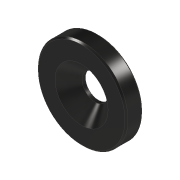
# Autodesk Inventor part: ring wiel
Saved by Autodesk Inventor 2020.3 (Build 243373000, 373)
## iProperties
Created: 2020-09-10
Part Number: ring wiel
Material: Stainless Steel
Document SubType Name: Modeling
Designer: Svend
Density: 8 g/cm^3
Appearance: Semi-Polished
Author: Svend
Autodesk Inventor part; units mm, degrees
ref_plane "YZ Plane" through (0, 0, 0) normal (1, 0, 0) x (0, 1, 0)
ref_plane "XZ Plane" through (0, 0, 0) normal (0, 1, 0) x (-1, 0, 0)
ref_plane "XY Plane" through (0, 0, 0) normal (0, 0, 1) x (1, 0, 0)
sketch "Sketch1" plane through (0, 0, 0) normal (0, 0, 1) x (1, 0, 0)
  circle A0 centre (0, 0) radius 14.65
  dimension "d0" = 29.3
  constraints: 1 centre point, 1 coincident
  measures "d0" diameter of A0
extrude "Extrusion1" add sketch "Sketch1" along normal blind 5.5
chamfer "Chamfer1" distance 0.5 angle 45 2 edges at (-14.65, 0, 5.5) (-14.65, 0, 0)
sketch "Sketch2" plane through (0, 0, 5.5) normal (0, 0, 1) x (1, 0, 0)
  circle A0 centre (0, 0) radius 14.65 projected
  constraints: 1 coincident
hole "Hole1" at (0, 0, 5.5) direction (0, 0, -1) diameter 8.5 depth 8 tip angle 118 countersink diameter 17.3 countersink angle 90
body "Solid1"
